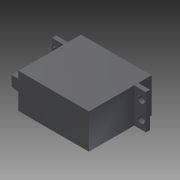
# Autodesk Inventor part: serwo HK15138
Saved by Autodesk Inventor 2013 (Build 170138000, 138)
## iProperties
Created: 2013-03-06
Part Number: serwo HK15138
Material: Generic
Document SubType Name: Modeling
Designer: Masta
Density: 1 g/cm^3
Author: Masta
Autodesk Inventor part; units mm, degrees
ref_plane "YZ Plane" through (0, 0, 0) normal (1, 0, 0) x (0, 1, 0)
ref_plane "XZ Plane" through (0, 0, 0) normal (0, 1, 0) x (-1, 0, 0)
ref_plane "XY Plane" through (0, 0, 0) normal (0, 0, 1) x (1, 0, 0)
sketch "Sketch1" plane through (0, 0, 0) normal (0, 1, 0) x (-1, 0, 0)
  line L0 (20.25, 10) -> (-20.25, 10)
  line L1 (-20.25, 10) -> (-20.25, -10)
  line L2 (-20.25, -10) -> (20.25, -10)
  line L3 (20.25, -10) -> (20.25, 10)
  line L4 (20.25, 10) -> (-20.25, -10) construction
  line L5 (-20.25, 10) -> (20.25, -10) construction
  line L6 (-27, 10) -> (-27, 6.25)
  line L7 (27, -10) -> (27, -6.25)
  line L8 (27, 10) -> (-27, -10) construction
  line L9 (-27, 10) -> (27, -10) construction
  line L10 (20.25, -10) -> (27, -10)
  line L11 (20.25, 10) -> (27, 10)
  line L12 (-20.25, 10) -> (-27, 10)
  line L13 (-20.25, -10) -> (-27, -10)
  line L14 (24.25, 5) -> (-24.25, 5) construction
  line L15 (-24.25, 5) -> (-24.25, -5) construction
  line L16 (-24.25, -5) -> (24.25, -5) construction
  line L17 (24.25, -5) -> (24.25, 5) construction
  line L18 (24.25, 5) -> (-24.25, -5) construction
  line L19 (-24.25, 5) -> (24.25, -5) construction
  circle A0 centre (-24.25, 5) radius 2
  line L20 (-27, 3.75) -> (-25.8112, 3.75)
  line L21 (-27, 6.25) -> (-25.8112, 6.25)
  line L22 (-20.25, 0) -> (20.25, 0) construction
  line L23 (0, 10) -> (0, -10) construction
  circle A1 centre (-24.25, -5) radius 2
  line L24 (-27, -3.75) -> (-25.8112, -3.75)
  line L25 (-27, -6.25) -> (-25.8112, -6.25)
  circle A2 centre (24.25, 5) radius 2
  line L26 (27, 3.75) -> (25.8112, 3.75)
  line L27 (27, 6.25) -> (25.8112, 6.25)
  line L28 (27, -6.25) -> (25.8112, -6.25)
  line L29 (27, -3.75) -> (25.8112, -3.75)
  circle A3 centre (24.25, -5) radius 2
  line L30 (-27, 3.75) -> (-27, -3.75)
  line L31 (-27, 6.25) -> (-27, 3.75)
  line L32 (-27, -6.25) -> (-27, -10)
  line L33 (-27, -3.75) -> (-27, -6.25)
  line L34 (27, -3.75) -> (27, 3.75)
  line L35 (27, -6.25) -> (27, -3.75)
  line L36 (27, 3.75) -> (27, 6.25)
  line L37 (27, 6.25) -> (27, 10)
  point P0 (0, 0)
  dimension "d0" = 40.5
  dimension "d1" = 20
  dimension "d2" = 54
  dimension "d3" = 48.5
  dimension "d4" = 10
  dimension "d12" = 2.5
  dimension "d13" = 4
  constraints: 76 end point, 32 parallel, 15 symmetric about line, 12 perpendicular, 10 midpoint, 8 point on circle, 4 centre point, 2 collinear, 2 horizontal, 1 coincident, 4 other
  measures "d0" distance of L2.end L1.end
  measures "d1" distance of L1.end L0.end
  measures "d2" distance of L7.start L8.end
  measures "d3" distance of L16.end L15.end
  measures "d4" distance of L15.end L14.end
  measures "d12" distance between parallel lines of L20 L21
  measures "d13" diameter of A0
extrude "Extrusion1" add sketch "Sketch1" along normal blind 10 and the other way blind 26 contours L3 L2 L1 L0
extrude "Extrusion2" add sketch "Sketch1" along normal blind 2.4 contours L11 L37 L27 A2 L26 L34 L29 A3 L28 L7 L10 L3 | L1 L13 L32 L25 A1 L24 L30 L20 A0 L21 L6 L12 | L36 L26 A2 L27 | L21 A0 L20 L31 | L28 A3 L29 L35 | L33 L24 A1 L25
sketch "Sketch2" plane through (0, 10, 0) normal (0, 1, 0) x (1, 0, 0)
  line L0 (-20.25, 10) -> (-20.25, -10) projected
  circle A0 centre (-10.25, 0) radius 6.5
  line L1 (-10.25, 0) -> (0, 0) construction
  dimension "d14" = 13
  dimension "d15" = 10
  constraints: 2 end point, 1 centre point, 1 perpendicular
  measures "d14" diameter of A0
  measures "d15" distance from line of L1.start L0
extrude "Extrusion3" add sketch "Sketch2" along normal blind 2
sketch "Sketch3" plane through (-10.25, 12, 0) normal (0, 1, 0) x (1, 0, 0)
  circle A0 centre (0, 0) radius 6.5 projected
  circle A1 centre (0, 0) radius 3
  point P0 (10.25, 0)
  dimension "d18" = 6
  constraints: 1 centre point, 1 coincident
  measures "d18" diameter of A1
extrude "Extrusion4" add sketch "Sketch3" along normal blind 4 contours A1
sketch "Sketch4" plane through (-20.25, -26, -10) normal (-1, 0, 0) x (0, 0, 1)
  line L0 (20, 26) -> (0, 26) projected
  line L1 (6.5, 2.5) -> (13.5, 2.5)
  line L2 (13.5, 2.5) -> (13.5, 7)
  line L3 (13.5, 7) -> (6.5, 7)
  line L4 (6.5, 7) -> (6.5, 2.5)
  line L5 (6.5, 2.5) -> (13.5, 7) construction
  line L6 (13.5, 2.5) -> (6.5, 7) construction
  line L7 (10, 26) -> (10, 4.75) construction
  dimension "d21" = 7
  dimension "d22" = 4.5
  dimension "d23" = 19
  constraints: 14 end point, 3 parallel, 2 midpoint, 1 horizontal, 1 perpendicular
  measures "d21" distance of L3.end L2.end
  measures "d22" distance of L2.end L1.end
  measures "d23" distance between parallel lines of L0 L3
extrude "Extrusion5" add sketch "Sketch4" along normal blind 7 draft -5
sketch "Sketch5" plane through (0, 0, 0) normal (0, 0, 1) x (1, 0, 0)
  line L0 (27, 2.4) -> (27, 0) projected
  line L1 (27, 0) -> (20.25, 0) projected
  line L2 (20.25, 0) -> (20.25, -26) projected
  line L3 (20.25, -26) -> (-20.25, -26) projected
  line L4 (-20.25, -26) -> (-20.25, -23.5) projected
  line L5 (-20.25, -23.5) -> (-27.25, -22.8876) projected
  line L6 (-27.25, -22.8876) -> (-27.25, -19.6124) projected
  line L7 (-27.25, -19.6124) -> (-20.25, -19) projected
  line L8 (-20.25, -19) -> (-20.25, 0) projected
  line L9 (-20.25, 0) -> (-27, 0) projected
  line L10 (-27, 0) -> (-27, 2.4) projected
  line L11 (-27, 2.4) -> (-20.25, 2.4) projected
  line L12 (-20.25, 2.4) -> (-20.25, 10) projected
  line L13 (-20.25, 10) -> (-16.75, 10) projected
  line L14 (-16.75, 10) -> (-16.75, 12) projected
  line L15 (-16.75, 12) -> (-13.25, 12) projected
  line L16 (-13.25, 12) -> (-13.25, 16) projected
  line L17 (-13.25, 16) -> (-7.25, 16) projected
  line L18 (-7.25, 16) -> (-7.25, 12) projected
  line L19 (-7.25, 12) -> (-3.75, 12) projected
  line L20 (-3.75, 12) -> (-3.75, 10) projected
  line L21 (-3.75, 10) -> (20.25, 10) projected
  line L22 (20.25, 10) -> (20.25, 2.4) projected
  line L23 (20.25, 2.4) -> (27, 2.4) projected
  line L24 (-27, 2.4) -> (-20.25, 3.5)
  line L25 (20.25, 3.5) -> (27, 2.4)
  point P0 (0, 0)
  dimension "d26" = 1.1
  constraints: 4 end point, 2 point on line, 1 equal length
  measures "d26" distance of L24.end L11.end
extrude "Extrusion6" add sketch "Sketch5" along normal mid plane 1.3 contours L23 L22 L25 | L24 L12 L11
sketch "Sketch6" plane through (0, 10, 0) normal (0, 1, 0) x (1, 0, 0)
  line L0 (14.396, -7.1292) -> (14.396, 6.9984) construction
  line L1 (14.396, 6.9984) -> (17.9697, 6.9984) construction
  line L2 (17.9697, 6.9984) -> (17.9697, -7.1292) construction
  line L3 (17.9697, -7.1292) -> (14.396, -7.1292) construction
  line L4 (16.9527, -5.0608) -> (16.9527, -5.393)
  line L5 (16.9527, -5.393) -> (15.729, -5.393)
  line L6 (15.729, -5.393) -> (15.729, -6.5437)
  line L7 (15.729, -6.5437) -> (16.9527, -6.5437)
  line L8 (16.9527, -6.5437) -> (16.9527, -6.876)
  line L9 (16.9527, -6.876) -> (14.4527, -6.876)
  line L10 (14.4527, -6.876) -> (14.4527, -6.5437)
  line L11 (14.4527, -6.5437) -> (15.4333, -6.5437)
  line L12 (15.4333, -6.5437) -> (15.4333, -5.393)
  line L13 (15.4333, -5.393) -> (14.4527, -5.393)
  line L14 (14.4527, -5.393) -> (14.4527, -5.0608)
  line L15 (14.4527, -5.0608) -> (16.9527, -5.0608)
  line L16 (16.9527, -2.7309) -> (16.9527, -3.1625)
  line L17 (16.9527, -3.1625) -> (15.7898, -4.0762)
  line L18 (15.7898, -4.0762) -> (15.9539, -4.222)
  line L19 (15.9539, -4.222) -> (16.9527, -4.222)
  line L20 (16.9527, -4.222) -> (16.9527, -4.5543)
  line L21 (16.9527, -4.5543) -> (14.4527, -4.5543)
  line L22 (14.4527, -4.5543) -> (14.4527, -4.222)
  line L23 (14.4527, -4.222) -> (15.6014, -4.222)
  line L24 (15.6014, -4.222) -> (14.4527, -3.1969)
  line L25 (14.4527, -3.1969) -> (14.4527, -2.7917)
  line L26 (14.4527, -2.7917) -> (15.569, -3.827)
  line L27 (15.569, -3.827) -> (16.9527, -2.7309)
  line L28 (16.9527, -1.1872) -> (16.9527, -2.4068)
  line L29 (16.9527, -2.4068) -> (16.6974, -2.4068)
  line L30 (16.6974, -2.4068) -> (16.6974, -1.953)
  line L31 (16.6974, -1.953) -> (15.022, -1.953)
  line L32 (15.022, -1.953) -> (15.022, -2.4068)
  line L33 (15.022, -2.4068) -> (14.7931, -2.4068)
  spline S0 degree 2 poles (14.7931, -2.4068) (14.7931, -2.1495) (14.6472, -1.9064) (14.4446, -1.8902) knots 0 0 0 1 2 2 2
  line L34 (14.4446, -1.8902) -> (14.4446, -1.6309)
  line L35 (14.4446, -1.6309) -> (16.6974, -1.6309)
  line L36 (16.6974, -1.6309) -> (16.6974, -1.1872)
  line L37 (16.6974, -1.1872) -> (16.9527, -1.1872)
  spline S1 degree 2 poles (16.1585, 0.7881) (16.3388, 0.7881) (16.6468, 0.6726) (16.7602, 0.5673) knots 0 0 0 1 2 2 2
  spline S2 degree 2 poles (16.7602, 0.5673) (16.8737, 0.4619) (17.0054, 0.1479) (17.0054, -0.0466) knots 0 0 0 1 2 2 2
  spline S3 degree 2 poles (17.0054, -0.0466) (17.0054, -0.2249) (16.9264, -0.5733) (16.8636, -0.701) knots 0 0 0 1 2 2 2
  line L38 (16.8636, -0.701) -> (16.509, -0.701)
  line L39 (16.509, -0.701) -> (16.509, -0.6766)
  spline S4 degree 2 poles (16.509, -0.6766) (16.5374, -0.6381) (16.6103, -0.4943) (16.6427, -0.4072) knots 0 0 0 1 2 2 2
  spline S5 degree 2 poles (16.6427, -0.4072) (16.6772, -0.3079) (16.7157, -0.1438) (16.7157, -0.0405) knots 0 0 0 1 2 2 2
  spline S6 degree 2 poles (16.7157, -0.0405) (16.7157, 0.0608) (16.6427, 0.2512) (16.5637, 0.3201) knots 0 0 0 1 2 2 2
  spline S7 degree 2 poles (16.5637, 0.3201) (16.4888, 0.3829) (16.2902, 0.4478) (16.1565, 0.4478) knots 0 0 0 1 2 2 2
  spline S8 degree 2 poles (16.1565, 0.4478) (16.0228, 0.4478) (15.8526, 0.3748) (15.7959, 0.3059) knots 0 0 0 1 2 2 2
  spline S9 degree 2 poles (15.7959, 0.3059) (15.7331, 0.235) (15.6804, 0.0243) (15.6804, -0.1033) knots 0 0 0 1 2 2 2
  spline S10 degree 2 poles (15.6804, -0.1033) (15.6804, -0.2411) (15.723, -0.5146) (15.7412, -0.5976) knots 0 0 0 1 2 2 2
  line L40 (15.7412, -0.5976) -> (14.4527, -0.5976)
  line L41 (14.4527, -0.5976) -> (14.4527, 0.7739)
  line L42 (14.4527, 0.7739) -> (14.7465, 0.7739)
  line L43 (14.7465, 0.7739) -> (14.7465, -0.2755)
  line L44 (14.7465, -0.2755) -> (15.413, -0.2755)
  spline S11 degree 2 poles (15.413, -0.2755) (15.4049, -0.2147) (15.3988, -0.0972) (15.3988, -0.0486) knots 0 0 0 1 2 2 2
  spline S12 degree 2 poles (15.3988, -0.0486) (15.3988, 0.1439) (15.4616, 0.4093) (15.5548, 0.5308) knots 0 0 0 1 2 2 2
  spline S13 degree 2 poles (15.5548, 0.5308) (15.648, 0.6544) (15.9316, 0.7881) (16.1585, 0.7881) knots 0 0 0 1 2 2 2
  line L45 (16.9527, 2.5649) -> (16.9527, 1.3452)
  line L46 (16.9527, 1.3452) -> (16.6974, 1.3452)
  line L47 (16.6974, 1.3452) -> (16.6974, 1.799)
  line L48 (16.6974, 1.799) -> (15.022, 1.799)
  line L49 (15.022, 1.799) -> (15.022, 1.3452)
  line L50 (15.022, 1.3452) -> (14.7931, 1.3452)
  spline S14 degree 2 poles (14.7931, 1.3452) (14.7931, 1.6025) (14.6472, 1.8456) (14.4446, 1.8619) knots 0 0 0 1 2 2 2
  line L51 (14.4446, 1.8619) -> (14.4446, 2.1212)
  line L52 (14.4446, 2.1212) -> (16.6974, 2.1212)
  line L53 (16.6974, 2.1212) -> (16.6974, 2.5649)
  line L54 (16.6974, 2.5649) -> (16.9527, 2.5649)
  spline S15 degree 2 poles (14.6897, 3.6994) (14.6897, 3.6082) (14.7343, 3.4279) (14.7687, 3.3408) knots 0 0 0 1 2 2 2
  spline S16 degree 2 poles (14.7687, 3.3408) (14.8032, 3.2597) (14.8761, 3.1402) (14.9085, 3.0936) knots 0 0 0 1 2 2 2
  line L55 (14.9085, 3.0936) -> (14.9085, 3.0734)
  line L56 (14.9085, 3.0734) -> (14.554, 3.0734)
  spline S17 degree 2 poles (14.554, 3.0734) (14.4952, 3.1828) (14.4, 3.5576) (14.4, 3.7257) knots 0 0 0 1 2 2 2
  spline S18 degree 2 poles (14.4, 3.7257) (14.4, 3.8959) (14.4689, 4.1491) (14.5418, 4.2525) knots 0 0 0 1 2 2 2
  spline S19 degree 2 poles (14.5418, 4.2525) (14.6209, 4.3619) (14.8498, 4.4753) (15.0038, 4.4753) knots 0 0 0 1 2 2 2
  spline S20 degree 2 poles (15.0038, 4.4753) (15.2104, 4.4753) (15.5224, 4.2038) (15.5629, 4.0134) knots 0 0 0 1 2 2 2
  line L57 (15.5629, 4.0134) -> (15.5872, 4.0134)
  spline S21 degree 2 poles (15.5872, 4.0134) (15.6034, 4.0924) (15.6764, 4.2727) (15.7493, 4.3497) knots 0 0 0 1 2 2 2
  spline S22 degree 2 poles (15.7493, 4.3497) (15.8202, 4.4267) (16.0471, 4.5239) (16.2112, 4.5239) knots 0 0 0 1 2 2 2
  spline S23 degree 2 poles (16.2112, 4.5239) (16.3794, 4.5239) (16.665, 4.4084) (16.7744, 4.3031) knots 0 0 0 1 2 2 2
  spline S24 degree 2 poles (16.7744, 4.3031) (16.8879, 4.1937) (17.0054, 3.8837) (17.0054, 3.6872) knots 0 0 0 1 2 2 2
  spline S25 degree 2 poles (17.0054, 3.6872) (17.0054, 3.4988) (16.9142, 3.1301) (16.8514, 3.0045) knots 0 0 0 1 2 2 2
  line L58 (16.8514, 3.0045) -> (16.4969, 3.0045)
  line L59 (16.4969, 3.0045) -> (16.4969, 3.0288)
  spline S26 degree 2 poles (16.4969, 3.0288) (16.5739, 3.1341) (16.7157, 3.4907) (16.7157, 3.667) knots 0 0 0 1 2 2 2
  spline S27 degree 2 poles (16.7157, 3.667) (16.7157, 3.7703) (16.6508, 3.9769) (16.5759, 4.0458) knots 0 0 0 1 2 2 2
  spline S28 degree 2 poles (16.5759, 4.0458) (16.5009, 4.1127) (16.3226, 4.1836) (16.1869, 4.1836) knots 0 0 0 1 2 2 2
  spline S29 degree 2 poles (16.1869, 4.1836) (16.0512, 4.1836) (15.8749, 4.1046) (15.8243, 4.0337) knots 0 0 0 1 2 2 2
  spline S30 degree 2 poles (15.8243, 4.0337) (15.7736, 3.9627) (15.7351, 3.7703) (15.7351, 3.6568) knots 0 0 0 1 2 2 2
  line L60 (15.7351, 3.6568) -> (15.7351, 3.515)
  line L61 (15.7351, 3.515) -> (15.4576, 3.515)
  line L62 (15.4576, 3.515) -> (15.4576, 3.6264)
  spline S31 degree 2 poles (15.4576, 3.6264) (15.4576, 3.8513) (15.2428, 4.1349) (15.0382, 4.1349) knots 0 0 0 1 2 2 2
  spline S32 degree 2 poles (15.0382, 4.1349) (14.943, 4.1349) (14.8072, 4.062) (14.7667, 4.0033) knots 0 0 0 1 2 2 2
  spline S33 degree 2 poles (14.7667, 4.0033) (14.7242, 3.9405) (14.6897, 3.7865) (14.6897, 3.6994) knots 0 0 0 1 2 2 2
  spline S34 degree 2 poles (17.0094, 5.6564) (17.0094, 5.47) (16.898, 5.1641) (16.7947, 5.0567) knots 0 0 0 1 2 2 2
  spline S35 degree 2 poles (16.7947, 5.0567) (16.6934, 4.9514) (16.4179, 4.842) (16.2619, 4.842) knots 0 0 0 1 2 2 2
  spline S36 degree 2 poles (16.2619, 4.842) (16.0593, 4.842) (15.7189, 5.0588) (15.6176, 5.2654) knots 0 0 0 1 2 2 2
  line L63 (15.6176, 5.2654) -> (15.6075, 5.2654)
  spline S37 degree 2 poles (15.6075, 5.2654) (15.5001, 5.0811) (15.2448, 4.9028) (15.0544, 4.9028) knots 0 0 0 1 2 2 2
  spline S38 degree 2 poles (15.0544, 4.9028) (14.7728, 4.9028) (14.396, 5.3282) (14.396, 5.6564) knots 0 0 0 1 2 2 2
  spline S39 degree 2 poles (14.396, 5.6564) (14.396, 5.9968) (14.7525, 6.408) (15.0321, 6.408) knots 0 0 0 1 2 2 2
  spline S40 degree 2 poles (15.0321, 6.408) (15.2003, 6.408) (15.5285, 6.2115) (15.6217, 6.0272) knots 0 0 0 1 2 2 2
  line L64 (15.6217, 6.0272) -> (15.6318, 6.0272)
  spline S41 degree 2 poles (15.6318, 6.0272) (15.7331, 6.246) (16.0248, 6.4708) (16.2558, 6.4708) knots 0 0 0 1 2 2 2
  spline S42 degree 2 poles (16.2558, 6.4708) (16.5759, 6.4708) (17.0094, 6.0049) (17.0094, 5.6564) knots 0 0 0 1 2 2 2
  spline S43 degree 2 poles (16.2882, 6.1264) (16.1342, 6.1264) (15.9519, 6.0049) (15.8587, 5.8327) knots 0 0 0 1 2 2 2
  spline S44 degree 2 poles (15.8587, 5.8327) (15.8263, 5.776) (15.7513, 5.5855) (15.7027, 5.466) knots 0 0 0 1 2 2 2
  spline S45 degree 2 poles (15.7027, 5.466) (15.7939, 5.3282) (16.0653, 5.1803) (16.2375, 5.1803) knots 0 0 0 1 2 2 2
  spline S46 degree 2 poles (16.2375, 5.1803) (16.4645, 5.1803) (16.7602, 5.4538) (16.7602, 5.6605) knots 0 0 0 1 2 2 2
  spline S47 degree 2 poles (16.7602, 5.6605) (16.7602, 5.8712) (16.507, 6.1264) (16.2882, 6.1264) knots 0 0 0 1 2 2 2
  spline S48 degree 2 poles (15.0362, 6.0798) (14.868, 6.0798) (14.6431, 5.855) (14.6431, 5.6544) knots 0 0 0 1 2 2 2
  spline S49 degree 2 poles (14.6431, 5.6544) (14.6431, 5.4721) (14.8437, 5.2391) (15.0159, 5.2391) knots 0 0 0 1 2 2 2
  spline S50 degree 2 poles (15.0159, 5.2391) (15.1395, 5.2391) (15.3117, 5.3586) (15.3806, 5.4781) knots 0 0 0 1 2 2 2
  spline S51 degree 2 poles (15.3806, 5.4781) (15.4089, 5.5288) (15.5082, 5.7435) (15.5366, 5.8307) knots 0 0 0 1 2 2 2
  spline S52 degree 2 poles (15.5366, 5.8307) (15.4251, 5.9765) (15.1881, 6.0798) (15.0362, 6.0798) knots 0 0 0 1 2 2 2
  point P0 (0, 0)
  constraints: 2 other
emboss "Emboss1" sketch "Sketch6" operation cut depth 0.1 direction (0, -1, 0)
hole "Hole1" at (-10.25, 16, 0) direction (0, -1, 0) diameter 2.459 depth 8 tip angle 118 thread size "M3x0.5" class "6H" standard "ISO Metric profile"
body "Solid1"
